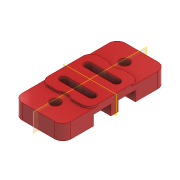
# Autodesk Inventor part: limit switch mount to xrail
Saved by Autodesk Inventor 2020 (Build 240168000, 168)
## iProperties
Created: 2019-11-26
Part Number: limit switch mount to xrail
Material: Generic
Document SubType Name: Modeling
Designer: ball
Density: 1 g/cm^3
Appearance: Default
Author: ball
Autodesk Inventor part; units mm, degrees
ref_plane "XZ Plane" through (0, 0, 0) normal (0, 1, 0) x (-1, 0, 0)
sketch "Sketch1" plane through (0, 0, 0) normal (0, 1, 0) x (-1, 0, 0)
  line L0 (-9.525, 20.1041) -> (9.525, 20.1041)
  line L1 (9.525, 20.1041) -> (9.525, -20.1041)
  line L2 (9.525, -20.1041) -> (-9.525, -20.1041)
  line L3 (-9.525, -20.1041) -> (-9.525, 20.1041)
  line L4 (-9.525, 20.1041) -> (9.525, -20.1041) construction
  line L5 (9.525, 20.1041) -> (-9.525, -20.1041) construction
  line L6 (-5.3594, 9.9441) -> (5.3594, 9.9441) construction
  line L7 (5.3594, 9.9441) -> (5.3594, -9.9441) construction
  line L8 (5.3594, -9.9441) -> (-5.3594, -9.9441) construction
  line L9 (-5.3594, -9.9441) -> (-5.3594, 9.9441) construction
  line L10 (-5.3594, 9.9441) -> (5.3594, -9.9441) construction
  line L11 (5.3594, 9.9441) -> (-5.3594, -9.9441) construction
  circle A0 centre (0, 13.4747) radius 1.9304
  circle A1 centre (0, 13.4747) radius 4.445 construction
  circle A2 centre (0, -13.4747) radius 1.9304
  circle A3 centre (0, -13.4747) radius 4.445 construction
  line L12 (9.525, 0) -> (-9.525, 0) construction
  point P0 (0, 0)
  dimension "d0" = 19.05
  dimension "d1" = 40.2082
  dimension "d2" = 10.7188
  dimension "d3" = 19.8882
  dimension "d5" = 3.8608
  dimension "d7" = 8.89
  dimension "d8" = 3.8608
  dimension "d10" = 8.89
  dimension "d33" = 26.9494
  constraints: 26 end point, 6 midpoint, 4 centre point, 4 parallel, 2 coincident, 2 horizontal, 2 perpendicular, 1 symmetric about line
  measures "d0" distance of L1.end L2.end
  measures "d1" distance of L0.end L1.end
  measures "d2" distance of L7.end L8.end
  measures "d3" distance of L6.end L7.end
  measures "d5" diameter of A0
  measures "d7" diameter of A1
  measures "d8" diameter of A2
  measures "d10" diameter of A3
  measures "d33" distance of A2.centre A0.centre
extrude "TNutMount" add sketch "Sketch1" along normal blind 5.9436
sketch "Sketch2" plane through (0, 5.9436, 0) normal (0, 1, 0) x (1, 0, 0)
  line L0 (-9.525, -9.9441) -> (9.525, -9.9441)
  line L1 (9.525, -9.9441) -> (9.525, 9.9441)
  line L2 (9.525, 9.9441) -> (-9.525, 9.9441)
  line L3 (-9.525, 9.9441) -> (-9.525, -9.9441)
  line L4 (-9.525, -9.9441) -> (9.525, 9.9441) construction
  line L5 (9.525, -9.9441) -> (-9.525, 9.9441) construction
  point P0 (0, 0)
  dimension "d13" = 19.05
  dimension "d14" = 19.8882
  constraints: 12 end point, 2 midpoint, 2 parallel, 1 horizontal, 1 perpendicular
  measures "d13" distance of L2.end L1.end
  measures "d14" distance of L1.end L0.end
extrude "SwitchMount" add sketch "Sketch2" along normal blind 0.6858
sketch "Sketch3" plane through (0, 6.6294, 0) normal (0, 1, 0) x (1, 0, 0)
  line L0 (5.588, -4.7625) -> (-5.588, -4.7625) construction
  line L1 (-5.588, -4.7625) -> (-5.588, 4.7625) construction
  line L2 (-5.588, 4.7625) -> (5.588, 4.7625) construction
  line L3 (5.588, 4.7625) -> (5.588, -4.7625) construction
  line L4 (5.588, -4.7625) -> (-5.588, 4.7625) construction
  line L5 (-5.588, -4.7625) -> (5.588, 4.7625) construction
  line L6 (-5.588, 4.7625) -> (5.588, 4.7625) construction
  line L7 (-5.588, 3.3528) -> (5.588, 3.3528)
  line L8 (5.588, 6.1722) -> (-5.588, 6.1722)
  arc A0 (-5.588, 6.1722) -> (-5.588, 3.3528) centre (-5.588, 4.7625) ccw
  arc A1 (5.588, 3.3528) -> (5.588, 6.1722) centre (5.588, 4.7625) ccw
  line L9 (-5.588, -4.7625) -> (5.588, -4.7625) construction
  line L10 (-5.588, -6.1722) -> (5.588, -6.1722)
  line L11 (5.588, -3.3528) -> (-5.588, -3.3528)
  arc A2 (-5.588, -3.3528) -> (-5.588, -6.1722) centre (-5.588, -4.7625) ccw
  arc A3 (5.588, -6.1722) -> (5.588, -3.3528) centre (5.588, -4.7625) ccw
  point P0 (0, 0)
  point P1 (0, 4.7625)
  point P2 (0, -4.7625)
  dimension "d19" = 11.176
  dimension "d20" = 9.525
  dimension "d21" = 2.8194
  dimension "d22" = 2.8194
  constraints: 28 end point, 8 point on circle, 8 tangent, 6 equal length, 4 centre point, 4 midpoint, 1 horizontal, 1 perpendicular
  measures "d19" distance of L1.end L2.end
  measures "d20" distance of L0.end L1.end
  measures "d21" diameter of A1
  measures "d22" diameter of A3
extrude "ScrewSlot" cut sketch "Sketch3" against normal through all
sketch "Sketch4" plane through (0, 0, 0) normal (0, -1, 0) x (1, 0, 0)
  arc A0 (5.588, -6.1722) -> (5.588, -3.3528) centre (5.588, -4.7625) ccw projected
  arc A1 (-5.588, -3.3528) -> (-5.588, -6.1722) centre (-5.588, -4.7625) ccw projected
  line L0 (5.588, -4.7625) -> (-5.588, -4.7625) construction
  arc A2 (5.588, 3.3528) -> (5.588, 6.1722) centre (5.588, 4.7625) ccw construction
  arc A3 (-5.588, 6.1722) -> (-5.588, 3.3528) centre (-5.588, 4.7625) ccw construction
  line L1 (5.588, 4.7625) -> (-5.588, 4.7625) construction
  line L2 (-9.525, -1.397) -> (9.525, -1.397)
  line L3 (9.525, -1.397) -> (9.525, -8.128)
  line L4 (9.525, -8.128) -> (-9.525, -8.128)
  line L5 (-9.525, -8.128) -> (-9.525, -1.397)
  line L6 (-9.525, -1.397) -> (9.525, -8.128) construction
  line L7 (9.525, -1.397) -> (-9.525, -8.128) construction
  line L8 (-9.525, 8.128) -> (9.525, 8.128)
  line L9 (9.525, 8.128) -> (9.525, 1.397)
  line L10 (9.525, 1.397) -> (-9.525, 1.397)
  line L11 (-9.525, 1.397) -> (-9.525, 8.128)
  line L12 (-9.525, 8.128) -> (9.525, 1.397) construction
  line L13 (9.525, 8.128) -> (-9.525, 1.397) construction
  point P0 (0, 0)
  point P1 (0, -4.7625)
  point P2 (0, 4.7625)
  dimension "d25" = 19.05
  dimension "d26" = 6.731
  dimension "d27" = 19.05
  dimension "d28" = 6.731
  constraints: 28 end point, 6 midpoint, 4 horizontal, 4 parallel, 2 perpendicular
  measures "d25" distance of L3.end L4.end
  measures "d26" distance of L2.end L3.end
  measures "d27" distance of L9.end L10.end
  measures "d28" distance of L8.end L9.end
extrude "Extrusion4" cut sketch "Sketch4" against normal blind 3.937
fillet "Fillet1" radius 3.175 8 edges at (9.525, 2.9718, 20.1041) (9.525, 2.9718, -20.1041) (-9.525, 2.9718, 20.1041) (-9.525, 2.9718, -20.1041) (9.525, 6.2865, -9.9441) (9.525, 6.2865, 9.9441) (-9.525, 6.2865, -9.9441) (-9.525, 6.2865, 9.9441)
sketch "Sketch5" plane through (0, 5.9436, 0) normal (0, 1, 0) x (1, 0, 0)
  circle A0 centre (0, 13.4747) radius 1.9304 projected
  circle A1 centre (0, 13.4747) radius 4.445
  circle A2 centre (0, -13.4747) radius 1.9304 projected
  circle A3 centre (0, -13.4747) radius 4.445
  point P0 (0, 0)
  dimension "d36" = 8.89
  dimension "d37" = 8.89
  constraints: 2 centre point, 2 coincident
  measures "d36" diameter of A1
  measures "d37" diameter of A3
extrude "Extrusion5" cut sketch "Sketch5" along normal up to surface (0.6858 mm away)
body "Solid1"
